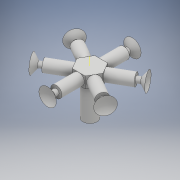
# Autodesk Inventor part: 武士刀夾具
Saved by Autodesk Inventor 2017 (Build 210142000, 142)
## iProperties
Created: 2021-05-18
Part Number: 武士刀夾具
Material: Generic
Document SubType Name: Modeling
Designer: user
Density: 1 g/cm^3
Appearance: Default
Author: user
Autodesk Inventor part; units mm, degrees
ref_plane "YZ Plane" through (0, 0, 0) normal (1, 0, 0) x (0, 1, 0)
ref_plane "XZ Plane" through (0, 0, 0) normal (0, 1, 0) x (-1, 0, 0)
ref_plane "XY Plane" through (0, 0, 0) normal (0, 0, 1) x (1, 0, 0)
sketch "Sketch1" plane through (0, 0, 0) normal (0, 0, 1) x (1, 0, 0)
  circle A0 centre (0, 0) radius 25
  dimension "d0" = 50
  constraints: 1 centre point, 1 coincident
  measures "d0" diameter of A0
extrude "Extrusion1" add sketch "Sketch1" along normal blind 120
sketch "Sketch2" plane through (0, 0, 120) normal (0, 0, 1) x (1, 0, 0)
  line L0 (46.188, 0) -> (23.094, -40)
  line L1 (23.094, -40) -> (-23.094, -40)
  line L2 (-23.094, -40) -> (-46.188, 0)
  line L3 (-46.188, 0) -> (-23.094, 40)
  line L4 (-23.094, 40) -> (23.094, 40)
  line L5 (23.094, 40) -> (46.188, 0)
  point P0 (0, 0)
  point P1 (0, 0)
  dimension "d4" = 40
  constraints: 12 end point, 1 coincident, 13 other
  measures "d4" distance from line of point (0, 0) L4
extrude "Extrusion2" add sketch "Sketch2" along normal blind 40 separate body
sketch "Sketch3" plane through (-23.094, 40, 120) normal (0, 1, 0) x (1, 0, 0)
  line L0 (0, 0) -> (0, -40) projected
  line L1 (0, -20) -> (46.188, -20)
  line L2 (46.188, 0) -> (46.188, -40) projected
  circle A0 centre (23.094, -20) radius 20
  point P0 (23.094, 120)
  constraints: 3 midpoint, 2 end point, 1 centre point
extrude "Extrusion3" add sketch "Sketch3" along normal blind 80 separate body
ref_plane "Work Plane1" through (0, 40, 140) normal (-1, 0, 0) x (0, 1, 0)
sketch "Sketch4" plane through (0, 40, 140) normal (-1, 0, 0) x (0, 1, 0)
  arc A0 (100, 0) -> (110.6837, -30.8906) centre (150, 0) ccw
  line L0 (0, 20) -> (0, -20) projected
  line L1 (150, 0) -> (0, 0)
  line L2 (110.6837, -30.8906) -> (94.27, -10)
  line L3 (94.27, -10) -> (80, -10)
  line L4 (80, -20) -> (80, 20) projected
  line L5 (100, 0) -> (80, 0)
  line L6 (80, 0) -> (80, -10)
  line L7 (-126, 0) -> (196, 0) projected
  point P0 (-40, 140)
  point P1 (100.0097, -0.9845)
  dimension "d11" = 150
  dimension "d12" = 10
  constraints: 10 end point, 3 point on circle, 2 horizontal, 2 midpoint, 2 point on line, 1 centre point, 1 tangent, 1 vertical
  measures "d11" distance from line of L0 L1.start
  measures "d12" distance between parallel lines of L5 L3
revolve "Revolution1" add sketch "Sketch4" angle 360 about axis through (0, 40, 140) along (0, 1, 0) bodies 3
pattern_circular "Circular Pattern1" count 6 over 360 about axis through (0, 0, 0) along (0, 0, 1) bodies 3
ref_plane "Work Plane2" through (0, 0, 0) normal (0.8660254, 0.5, 0) x (0, 0, 1)
ref_plane "Work Plane3" through (0, 0, 0) normal (-0.5, -0.8660254, 0) x (0, 0, 1)
ref_plane "Work Plane4" through (-23.094, -40, 120) normal (-0.8660254, 0.5, 0) x (0, 0, 1)
body "Solid1"
body "Solid2"
body "Solid3"
body "Solid4"
body "Solid5"
body "Solid6"
body "Solid7"
body "Solid8"
